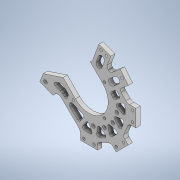
# Autodesk Inventor part: motor_holder_4
Saved by Autodesk Inventor 2020 (Build 240168000, 168)
## iProperties
Created: 2020-03-26
Part Number: motor_holder_4
Material: Generic
Document SubType Name: Modeling
Designer: psrobotics
Density: 1 g/cm^3
Appearance: Default
Author: psrobotics
Autodesk Inventor part; units mm, degrees
(part 1 of 2)
ref_plane "YZ Plane" through (0, 0, 0) normal (1, 0, 0) x (0, 1, 0)
ref_plane "XZ Plane" through (0, 0, 0) normal (0, 1, 0) x (-1, 0, 0)
ref_plane "XY Plane" through (0, 0, 0) normal (0, 0, 1) x (1, 0, 0)
sketch "Sketch1" plane through (0, 0, 0) normal (0, 0, 1) x (1, 0, 0)
  circle A0 centre (-20.1972, 20.1972) radius 3.075 projected
  arc A1 (-10.1972, -33.3775) -> (10.6148, -24.7569) centre (-20.1972, 20.1972) ccw projected
  arc A2 (-70.4, 41.4086) -> (-73.6451, 30.854) centre (-20.1972, 20.1972) ccw projected
  circle A3 centre (-68.634, 68.634) radius 50 projected
  circle A4 centre (-20.1972, 20.1972) radius 54.5
  circle A5 centre (-20.1972, 20.1972) radius 22.5
  circle A6 centre (-68.634, 68.634) radius 53
  point P0 (0, 0)
  point P1 (-15.9632, 74.5325)
  point P2 (-22.4794, 42.5811)
  point P3 (-42.5811, 22.4794)
  point P4 (-74.5325, 15.9632)
  point P5 (-73.6451, 30.854)
  point P6 (-10.1972, -33.3775)
  point P7 (10.6148, -24.7569)
  point P8 (-74.5325, 15.9632)
  dimension "d0" = 109
  dimension "d1" = 45
  dimension "d2" = 106
  constraints: 3 centre point, 3 coincident
  measures "d0" diameter of A4
  measures "d1" diameter of A5
  measures "d2" diameter of A6
extrude "Extrusion1" add sketch "Sketch1" along normal blind 5 contours A0 | A4 A6 A5 A1 | A6 A5
sketch "Sketch2" plane through (0, 0, 5) normal (0, 0, 1) x (1, 0, 0)
  arc A0 (-74.5325, 15.9632) -> (-15.9632, 74.5325) centre (-20.1972, 20.1972) ccw
  circle A1 centre (31.0318, 14.1972) radius 2.075
  circle A2 centre (-26.1972, -31.0318) radius 2.075
  circle A3 centre (-14.1972, -31.0318) radius 2.075
  circle A4 centre (31.0318, 26.1972) radius 2.075
  line L0 (34.8028, 30.1972) -> (27.2607, 30.1972)
  line L1 (27.2607, 10.1972) -> (27.2607, 30.1972)
  arc A5 (20.4317, -6.2895) -> (27.2607, 10.1972) centre (-20.1972, 20.1972) ccw
  line L2 (6.2895, -20.4317) -> (20.4317, -6.2895)
  arc A6 (-10.1972, -27.2607) -> (6.2895, -20.4317) centre (-20.1972, 20.1972) ccw
  line L3 (-30.1972, -27.2607) -> (-10.1972, -27.2607)
  line L4 (-30.1972, -27.2607) -> (-30.1972, -34.8028)
  line L5 (-10.1972, -34.8028) -> (-30.1972, -34.8028)
  line L6 (-10.1972, -33.3775) -> (-10.1972, -34.8028)
  arc A7 (-10.1972, -33.3775) -> (10.6148, -24.7569) centre (-20.1972, 20.1972) ccw
  line L7 (11.6226, -25.7648) -> (10.6148, -24.7569)
  line L8 (25.7648, -11.6226) -> (11.6226, -25.7648)
  line L9 (24.7569, -10.6148) -> (25.7648, -11.6226)
  arc A8 (24.7569, -10.6148) -> (33.3775, 10.1972) centre (-20.1972, 20.1972) ccw
  line L10 (34.8028, 10.1972) -> (33.3775, 10.1972)
  line L11 (34.8028, 30.1972) -> (34.8028, 10.1972)
  circle A9 centre (-10.8666, 70.4743) radius 2.075
  line L12 (-36.782, 65.7734) -> (-41.4086, 70.4)
  arc A10 (-17.5734, 68.6262) -> (-36.782, 65.7734) centre (-20.1972, 20.1972) ccw
  line L13 (-5.9823, 65.5203) -> (-17.5734, 68.6262)
  line L14 (-4.1597, 72.3225) -> (-5.9823, 65.5203)
  line L15 (-15.7508, 75.4283) -> (-4.1597, 72.3225)
  spline S0 degree 3 poles (-17.8978, 74.6487) (-17.5075, 74.6322) (-17.1177, 74.6921) (-16.3809, 74.9587) (-16.0413, 75.1637) (-15.7508, 75.4283) knots 0 0 0 0 0.498547 0.498547 1 1 1 1
  arc A11 (-17.8978, 74.6487) -> (-30.854, 73.6451) centre (-20.1972, 20.1972) ccw
  arc A12 (-30.854, 73.6451) -> (-41.4086, 70.4) centre (-20.1972, 20.1972) ccw
  circle A13 centre (-70.4743, 10.8666) radius 2.075
  line L16 (-70.4, 41.4086) -> (-65.7734, 36.782)
  arc A14 (-70.4, 41.4086) -> (-73.6451, 30.854) centre (-20.1972, 20.1972) ccw
  arc A15 (-73.6451, 30.854) -> (-74.6487, 17.8978) centre (-20.1972, 20.1972) ccw
  spline S1 degree 3 poles (-74.6487, 17.8978) (-74.6321, 17.5052) (-74.6928, 17.1132) (-74.9611, 16.377) (-75.1652, 16.0396) (-75.4283, 15.7508) knots 0 0 0 0 0.501453 0.501453 1 1 1 1
  line L17 (-72.3225, 4.1597) -> (-75.4283, 15.7508)
  line L18 (-65.5203, 5.9823) -> (-72.3225, 4.1597)
  line L19 (-68.6262, 17.5734) -> (-65.5203, 5.9823)
  arc A16 (-65.7734, 36.782) -> (-68.6262, 17.5734) centre (-20.1972, 20.1972) ccw
  line L20 (-75.4283, 15.7508) -> (-68.6262, 17.5734)
  line L21 (-15.7508, 75.4283) -> (-17.5734, 68.6262)
  point P0 (0, 0)
  constraints: 4 end point, 2 perpendicular, 1 other
extrude "Extrusion2" add sketch "Sketch2" against normal up to surface (5 mm away) contours A0 L4 L3 A6 L2 A5 L1 L0 | L6 L5 L4 A0 | A0 L9 L8 L7 | A0 L0 L11 L10 | L17 L20 L19 L18 A0 | A0 L18 L17 | L14 L13 L21 L15 A0 | A0 L15 L14 | A1 | A2 | A3 | A4
sketch "Sketch3" plane through (0, 0, 5) normal (0, 0, 1) x (1, 0, 0)
  circle A0 centre (31.0318, 26.1972) radius 2.075 projected
  circle A1 centre (31.0318, 14.1972) radius 2.075 projected
  circle A2 centre (-14.1972, -31.0318) radius 2.075 projected
  circle A3 centre (-26.1972, -31.0318) radius 2.075 projected
  circle A4 centre (-70.4743, 10.8666) radius 2.075 projected
  circle A5 centre (-10.8666, 70.4743) radius 2.075 projected
  point P0 (0, 0)
hole "Hole1" at (31.0318, 26.1972, 5) at (31.0318, 14.1972, 5) at (-14.1972, -31.0318, 5) at (-26.1972, -31.0318, 5) at (-70.4743, 10.8666, 5) at (-10.8666, 70.4743, 5) direction (0, 0, -1) diameter 4.15 depth 7
sketch "Sketch4" plane through (0, 0, 5) normal (0, 0, 1) x (1, 0, 0)
  circle A0 centre (-20.1972, 20.1972) radius 17.5 projected
  circle A1 centre (-20.1972, 20.1972) radius 22.5
  point P0 (0, 0)
  dimension "d14" = 45
  constraints: 1 centre point, 1 coincident
  measures "d14" diameter of A1
extrude "Extrusion3" cut sketch "Sketch4" against normal blind 10 contours A0 | A1
sketch "Sketch5" plane through (0, 0, 0) normal (0, 0, -1) x (-1, 0, 0)
  arc A0 (22.4794, 42.5811) -> (42.5811, 22.4794) centre (20.1972, 20.1972) ccw projected
  arc A1 (15.6366, 68.1072) -> (22.4794, 42.5811) centre (68.634, 68.634) ccw projected
  line L0 (15.6366, 68.1072) -> (17.5734, 68.6262) projected
  line L1 (17.5734, 68.6262) -> (15.7508, 75.4283) projected
  line L2 (15.7508, 75.4283) -> (4.1597, 72.3225) projected
  line L3 (4.1597, 72.3225) -> (4.1692, 72.287) projected
  arc A2 (4.1692, 72.287) -> (-33.3775, 30.1972) centre (20.1972, 20.1972) ccw projected
  line L4 (-33.3775, 30.1972) -> (-34.8028, 30.1972) projected
  line L5 (-34.8028, 30.1972) -> (-34.8028, 10.1972) projected
  line L6 (-34.8028, 10.1972) -> (-33.3775, 10.1972) projected
  arc A3 (-33.3775, 10.1972) -> (-24.7569, -10.6148) centre (20.1972, 20.1972) ccw projected
  line L7 (-24.7569, -10.6148) -> (-25.7648, -11.6226) projected
  line L8 (-25.7648, -11.6226) -> (-11.6226, -25.7648) projected
  line L9 (-11.6226, -25.7648) -> (-10.6148, -24.7569) projected
  arc A4 (-10.6148, -24.7569) -> (10.1972, -33.3775) centre (20.1972, 20.1972) ccw projected
  line L10 (10.1972, -33.3775) -> (10.1972, -34.8028) projected
  line L11 (10.1972, -34.8028) -> (30.1972, -34.8028) projected
  line L12 (30.1972, -34.8028) -> (30.1972, -33.3775) projected
  arc A5 (30.1972, -33.3775) -> (72.287, 4.1692) centre (20.1972, 20.1972) ccw projected
  line L13 (72.287, 4.1692) -> (72.3225, 4.1597) projected
  line L14 (72.3225, 4.1597) -> (75.4283, 15.7508) projected
  line L15 (75.4283, 15.7508) -> (68.6262, 17.5734) projected
  line L16 (68.6262, 17.5734) -> (68.1072, 15.6366) projected
  arc A6 (42.5811, 22.4794) -> (68.1072, 15.6366) centre (68.634, 68.634) ccw projected
  circle A7 centre (70.4743, 10.8666) radius 2.075 projected
  circle A8 centre (14.1972, -31.0318) radius 2.075 projected
  circle A9 centre (-31.0318, 26.1972) radius 2.075 projected
  circle A10 centre (-31.0318, 14.1972) radius 2.075 projected
  circle A11 centre (26.1972, -31.0318) radius 2.075 projected
  circle A12 centre (10.8666, 70.4743) radius 2.075 projected
  line L17 (72.3225, 4.1597) -> (65.5203, 5.9823) projected
  line L18 (30.1972, -34.8028) -> (30.1972, -5.9562) projected
  line L19 (-5.9562, 30.1972) -> (-34.8028, 30.1972) projected
  line L20 (4.1597, 72.3225) -> (5.9823, 65.5203) projected
  line L21 (20.1972, 20.1972) -> (0, 0)
  line L22 (5.9823, 65.5203) -> (-29.3408, 30.1972)
  line L23 (65.5203, 5.9823) -> (30.1972, -29.3408)
  constraints: 6 end point, 2 parallel, 2 point on line
extrude "Extrusion4" cut sketch "Sketch5" against normal blind 10 contours L20 L22 L19 A2 | A5 L18 L23 L17
sketch "Sketch6" plane through (0, 0, 5) normal (0, 0, 1) x (1, 0, 0)
  circle A0 centre (-70.4743, 10.8666) radius 2.075 projected
  circle A1 centre (-14.1972, -31.0318) radius 2.075 projected
  circle A2 centre (31.0318, 26.1972) radius 2.075 projected
  circle A3 centre (31.0318, 14.1972) radius 2.075 projected
  circle A4 centre (-26.1972, -31.0318) radius 2.075 projected
  circle A5 centre (-10.8666, 70.4743) radius 2.075 projected
  line L0 (34.8028, 30.1972) -> (29.3408, 30.1972) projected
  line L1 (29.3408, 30.1972) -> (-5.9823, 65.5203) projected
  line L2 (-5.9823, 65.5203) -> (-4.1597, 72.3225) projected
  line L3 (-4.1597, 72.3225) -> (-15.7508, 75.4283) projected
  line L4 (-15.7508, 75.4283) -> (-17.5734, 68.6262) projected
  line L5 (-17.5734, 68.6262) -> (-15.6366, 68.1072) projected
  arc A6 (-22.4794, 42.5811) -> (-15.6366, 68.1072) centre (-68.634, 68.634) ccw projected
  arc A7 (-42.5811, 22.4794) -> (-22.4794, 42.5811) centre (-20.1972, 20.1972) ccw projected
  arc A8 (-68.1072, 15.6366) -> (-42.5811, 22.4794) centre (-68.634, 68.634) ccw projected
  line L6 (-68.1072, 15.6366) -> (-68.6262, 17.5734) projected
  line L7 (-68.6262, 17.5734) -> (-75.4283, 15.7508) projected
  line L8 (-75.4283, 15.7508) -> (-72.3225, 4.1597) projected
  line L9 (-72.3225, 4.1597) -> (-65.5203, 5.9823) projected
  line L10 (-65.5203, 5.9823) -> (-30.1972, -29.3408) projected
  line L11 (-30.1972, -29.3408) -> (-30.1972, -34.8028) projected
  line L12 (-30.1972, -34.8028) -> (-10.1972, -34.8028) projected
  line L13 (-10.1972, -34.8028) -> (-10.1972, -33.3775) projected
  arc A9 (-10.1972, -33.3775) -> (10.6148, -24.7569) centre (-20.1972, 20.1972) ccw projected
  line L14 (10.6148, -24.7569) -> (11.6226, -25.7648) projected
  line L15 (11.6226, -25.7648) -> (25.7648, -11.6226) projected
  line L16 (25.7648, -11.6226) -> (24.7569, -10.6148) projected
  arc A10 (24.7569, -10.6148) -> (33.3775, 10.1972) centre (-20.1972, 20.1972) ccw projected
  line L17 (33.3775, 10.1972) -> (34.8028, 10.1972) projected
  line L18 (34.8028, 10.1972) -> (34.8028, 30.1972) projected
  line L19 (-20.1972, 20.1972) -> (-4.2873, 36.1071)
  arc A11 (-42.5811, 22.4794) -> (-22.4794, 42.5811) centre (-20.1972, 20.1972) ccw projected
  line L20 (-20.1972, 20.1972) -> (-36.1071, 4.2873)
  line L21 (-20.1972, 20.1972) -> (0, 0)
  line L22 (-4.2873, 36.1071) -> (-18.7922, 50.612)
  line L23 (-36.1071, 4.2873) -> (-50.612, 18.7922)
  point P0 (-36.1071, 4.2873)
  point P1 (-4.2873, 36.1071)
  constraints: 10 end point, 4 perpendicular, 4 point on circle
extrude "Extrusion5" cut sketch "Sketch6" against normal blind 10 contours L22 A7 A6 | L23 A8 A7
sketch "Sketch7" plane through (0, 0, 5) normal (0, 0, 1) x (1, 0, 0)
  circle A0 centre (-10.8666, 70.4743) radius 2.075 projected
  circle A1 centre (-26.1972, -31.0318) radius 2.075 projected
  circle A2 centre (31.0318, 14.1972) radius 2.075 projected
  circle A3 centre (31.0318, 26.1972) radius 2.075 projected
  circle A4 centre (-14.1972, -31.0318) radius 2.075 projected
  circle A5 centre (-70.4743, 10.8666) radius 2.075 projected
  line L0 (-36.1071, 4.2873) -> (-50.612, 18.7922) projected
  arc A6 (-68.1072, 15.6366) -> (-50.612, 18.7922) centre (-68.634, 68.634) ccw projected
  line L1 (-68.1072, 15.6366) -> (-68.6262, 17.5734) projected
  line L2 (-68.6262, 17.5734) -> (-75.4283, 15.7508) projected
  line L3 (-75.4283, 15.7508) -> (-72.3225, 4.1597) projected
  line L4 (-72.3225, 4.1597) -> (-65.5203, 5.9823) projected
  line L5 (-65.5203, 5.9823) -> (-30.1972, -29.3408) projected
  line L6 (-30.1972, -29.3408) -> (-30.1972, -34.8028) projected
  line L7 (-30.1972, -34.8028) -> (-10.1972, -34.8028) projected
  line L8 (-10.1972, -34.8028) -> (-10.1972, -33.3775) projected
  arc A7 (-10.1972, -33.3775) -> (10.6148, -24.7569) centre (-20.1972, 20.1972) ccw projected
  line L9 (10.6148, -24.7569) -> (11.6226, -25.7648) projected
  line L10 (11.6226, -25.7648) -> (25.7648, -11.6226) projected
  line L11 (25.7648, -11.6226) -> (24.7569, -10.6148) projected
  arc A8 (24.7569, -10.6148) -> (33.3775, 10.1972) centre (-20.1972, 20.1972) ccw projected
  line L12 (33.3775, 10.1972) -> (34.8028, 10.1972) projected
  line L13 (34.8028, 10.1972) -> (34.8028, 30.1972) projected
  line L14 (34.8028, 30.1972) -> (29.3408, 30.1972) projected
  line L15 (29.3408, 30.1972) -> (-5.9823, 65.5203) projected
  line L16 (-5.9823, 65.5203) -> (-4.1597, 72.3225) projected
  line L17 (-4.1597, 72.3225) -> (-15.7508, 75.4283) projected
  line L18 (-15.7508, 75.4283) -> (-17.5734, 68.6262) projected
  line L19 (-17.5734, 68.6262) -> (-15.6366, 68.1072) projected
  arc A9 (-18.7922, 50.612) -> (-15.6366, 68.1072) centre (-68.634, 68.634) ccw projected
  line L20 (-18.7922, 50.612) -> (-4.2873, 36.1071) projected
  arc A10 (-36.1071, 4.2873) -> (-4.2873, 36.1071) centre (-20.1972, 20.1972) ccw projected
  line L21 (-4.1597, 72.3225) -> (-5.9823, 65.5203) projected
  line L22 (-4.1597, 72.3225) -> (34.8028, 30.1972)
  line L23 (-72.3225, 4.1597) -> (-30.1972, -34.8028)
  point P0 (0, 0)
  constraints: 4 end point
extrude "Extrusion6" add sketch "Sketch7" against normal up to surface (5 mm away) contours L4 L5 L6 L23 | L22 L14 L15 L16
sketch "Sketch8" plane through (0, 0, 5) normal (0, 0, 1) x (1, 0, 0)
  circle A0 centre (31.0318, 14.1972) radius 2.075 projected
  circle A1 centre (31.0318, 26.1972) radius 2.075 projected
  circle A2 centre (-10.8666, 70.4743) radius 2.075 projected
  circle A3 centre (-70.4743, 10.8666) radius 2.075 projected
  circle A4 centre (-26.1972, -31.0318) radius 2.075 projected
  circle A5 centre (-14.1972, -31.0318) radius 2.075 projected
  circle A6 centre (-14.1972, -31.0318) radius 2.075 projected
  circle A7 centre (-14.1972, -31.0318) radius 1.5
  circle A8 centre (-26.1972, -31.0318) radius 2.075 projected
  circle A9 centre (-26.1972, -31.0318) radius 1.5
  circle A10 centre (-70.4743, 10.8666) radius 2.075 projected
  circle A11 centre (-70.4743, 10.8666) radius 1.5
  circle A12 centre (31.0318, 14.1972) radius 2.075 projected
  circle A13 centre (31.0318, 14.1972) radius 1.5
  circle A14 centre (31.0318, 26.1972) radius 2.075 projected
  circle A15 centre (31.0318, 26.1972) radius 1.5
  circle A16 centre (-10.8666, 70.4743) radius 2.075 projected
  circle A17 centre (-10.8666, 70.4743) radius 1.5
  point P0 (0, 0)
  dimension "d24" = 3
  dimension "d25" = 3
  dimension "d26" = 3
  dimension "d27" = 3
  dimension "d28" = 3
  dimension "d29" = 3
  constraints: 6 centre point, 6 coincident
  measures "d24" diameter of A7
  measures "d25" diameter of A9
  measures "d26" diameter of A11
  measures "d27" diameter of A13
  measures "d28" diameter of A15
  measures "d29" diameter of A17
extrude "Extrusion7" add sketch "Sketch8" against normal up to surface (5 mm away)
sketch "Sketch9" plane through (0, 0, 5) normal (0, 0, 1) x (1, 0, 0)
  circle A0 centre (-70.4743, 10.8666) radius 1.5 projected
  circle A1 centre (-14.1972, -31.0318) radius 1.5 projected
  circle A2 centre (31.0318, 26.1972) radius 1.5 projected
  circle A3 centre (31.0318, 14.1972) radius 1.5 projected
  circle A4 centre (-26.1972, -31.0318) radius 1.5 projected
  circle A5 centre (-10.8666, 70.4743) radius 1.5 projected
  line L0 (-36.1071, 4.2873) -> (-50.612, 18.7922) projected
  arc A6 (-68.1072, 15.6366) -> (-50.612, 18.7922) centre (-68.634, 68.634) ccw projected
  line L1 (-68.6262, 17.5734) -> (-75.4283, 15.7508) projected
  line L2 (-75.4283, 15.7508) -> (-72.3225, 4.1597) projected
  line L3 (-72.3225, 4.1597) -> (-30.1972, -34.8028) projected
  line L4 (-30.1972, -34.8028) -> (-10.1972, -34.8028) projected
  line L5 (-10.1972, -34.8028) -> (-10.1972, -33.3775) projected
  arc A7 (-10.1972, -33.3775) -> (10.6148, -24.7569) centre (-20.1972, 20.1972) ccw projected
  line L6 (10.6148, -24.7569) -> (11.6226, -25.7648) projected
  line L7 (11.6226, -25.7648) -> (25.7648, -11.6226) projected
  line L8 (25.7648, -11.6226) -> (24.7569, -10.6148) projected
  arc A8 (24.7569, -10.6148) -> (33.3775, 10.1972) centre (-20.1972, 20.1972) ccw projected
  line L9 (33.3775, 10.1972) -> (34.8028, 10.1972) projected
  line L10 (34.8028, 10.1972) -> (34.8028, 30.1972) projected
  line L11 (34.8028, 30.1972) -> (-4.1597, 72.3225) projected
  line L12 (-4.1597, 72.3225) -> (-15.7508, 75.4283) projected
  line L13 (-15.7508, 75.4283) -> (-17.5734, 68.6262) projected
  arc A9 (-18.7922, 50.612) -> (-15.6366, 68.1072) centre (-68.634, 68.634) ccw projected
  line L14 (-18.7922, 50.612) -> (-4.2873, 36.1071) projected
  arc A10 (-36.1071, 4.2873) -> (-4.2873, 36.1071) centre (-20.1972, 20.1972) ccw projected
  circle A11 centre (20.2698, -11.7845) radius 2.075 projected
  circle A12 centre (11.7845, -20.2698) radius 2.075 projected
  line L15 (-68.1072, 15.6366) -> (-68.6262, 17.5734) projected
  line L16 (-17.5734, 68.6262) -> (-15.6366, 68.1072) projected
  point P0 (0, 0)
hole "Hole2" at (20.2698, -11.7845, 5) at (11.7845, -20.2698, 5) direction (0, 0, -1) diameter 3 depth 7
sketch "Sketch10" plane through (0, 0, 5) normal (0, 0, 1) x (1, 0, 0)
  circle A0 centre (20.2698, -11.7845) radius 1.5 projected
  circle A1 centre (11.7845, -20.2698) radius 1.5 projected
  circle A2 centre (-70.4743, 10.8666) radius 1.5 projected
  circle A3 centre (-14.1972, -31.0318) radius 1.5 projected
  circle A4 centre (31.0318, 26.1972) radius 1.5 projected
  circle A5 centre (31.0318, 14.1972) radius 1.5 projected
  circle A6 centre (-26.1972, -31.0318) radius 1.5 projected
  circle A7 centre (-10.8666, 70.4743) radius 1.5 projected
  line L0 (-36.1071, 4.2873) -> (-50.612, 18.7922) projected
  arc A8 (-68.1072, 15.6366) -> (-50.612, 18.7922) centre (-68.634, 68.634) ccw projected
  line L1 (-68.6262, 17.5734) -> (-75.4283, 15.7508) projected
  line L2 (-75.4283, 15.7508) -> (-72.3225, 4.1597) projected
  line L3 (-72.3225, 4.1597) -> (-30.1972, -34.8028) projected
  line L4 (-30.1972, -34.8028) -> (-10.1972, -34.8028) projected
  line L5 (-10.1972, -34.8028) -> (-10.1972, -33.3775) projected
  arc A9 (-10.1972, -33.3775) -> (10.6148, -24.7569) centre (-20.1972, 20.1972) ccw projected
  line L6 (10.6148, -24.7569) -> (11.6226, -25.7648) projected
  line L7 (11.6226, -25.7648) -> (25.7648, -11.6226) projected
  line L8 (25.7648, -11.6226) -> (24.7569, -10.6148) projected
  arc A10 (24.7569, -10.6148) -> (33.3775, 10.1972) centre (-20.1972, 20.1972) ccw projected
  line L9 (33.3775, 10.1972) -> (34.8028, 10.1972) projected
  line L10 (34.8028, 10.1972) -> (34.8028, 30.1972) projected
  line L11 (34.8028, 30.1972) -> (-4.1597, 72.3225) projected
  line L12 (-4.1597, 72.3225) -> (-15.7508, 75.4283) projected
  line L13 (-15.7508, 75.4283) -> (-17.5734, 68.6262) projected
  arc A11 (-18.7922, 50.612) -> (-15.6366, 68.1072) centre (-68.634, 68.634) ccw projected
  line L14 (-18.7922, 50.612) -> (-4.2873, 36.1071) projected
  arc A12 (-36.1071, 4.2873) -> (-4.2873, 36.1071) centre (-20.1972, 20.1972) ccw projected
  line L15 (33.3775, 10.1972) -> (26.3775, 10.1972)
  line L16 (24.7569, -10.6148) -> (19.8072, -5.665)
  arc A13 (-10.1972, -33.3775) -> (10.6148, -24.7569) centre (-20.1972, 20.1972) ccw projected
  line L17 (10.6148, -24.7569) -> (5.665, -19.8072)
  line L18 (-10.1972, -33.3775) -> (-10.1972, -26.3775)
  line L19 (10.6148, -24.7569) -> (11.6226, -25.7648) projected
  line L20 (26.3775, 10.1972) -> (19.8072, -5.665)
  line L21 (5.665, -19.8072) -> (-10.1972, -26.3775)
  line L22 (-68.1072, 15.6366) -> (-68.6262, 17.5734) projected
  line L23 (-17.5734, 68.6262) -> (-15.6366, 68.1072) projected
  point P0 (0, 0)
  dimension "d39" = 7
  dimension "d40" = 7
  dimension "d41" = 7
  dimension "d42" = 7
  constraints: 12 end point, 2 collinear, 1 horizontal, 1 vertical
  measures "d39" distance of L9.start L15.end
  measures "d40" distance of L8.end L16.end
  measures "d41" distance of L6.start L17.end
  measures "d42" distance of L5.end L18.end
extrude "Extrusion8" cut sketch "Sketch10" against normal blind 10 contours L18 L21 L17 A9 | A10 L16 L20 L15
sketch "Sketch11" plane through (0, 0, 5) normal (0, 0, 1) x (1, 0, 0)
  line L0 (5.665, -19.8072) -> (11.6226, -25.7648) projected
  line L1 (11.6226, -25.7648) -> (25.7648, -11.6226) projected
  line L2 (25.7648, -11.6226) -> (19.8072, -5.665) projected
  line L3 (19.8072, -5.665) -> (26.3775, 10.1972) projected
  line L4 (26.3775, 10.1972) -> (34.8028, 10.1972) projected
  line L5 (34.8028, 10.1972) -> (34.8028, 30.1972) projected
  line L6 (34.8028, 30.1972) -> (-4.1597, 72.3225) projected
  line L7 (-4.1597, 72.3225) -> (-15.7508, 75.4283) projected
  line L8 (-15.7508, 75.4283) -> (-17.5734, 68.6262) projected
  arc A0 (-68.1072, 15.6366) -> (-50.612, 18.7922) centre (-68.634, 68.634) ccw projected
  line L9 (-18.7922, 50.612) -> (-4.2873, 36.1071) projected
  arc A1 (-36.1071, 4.2873) -> (-4.2873, 36.1071) centre (-20.1972, 20.1972) ccw projected
  line L10 (-36.1071, 4.2873) -> (-50.612, 18.7922) projected
  arc A2 (-18.7922, 50.612) -> (-15.6366, 68.1072) centre (-68.634, 68.634) ccw projected
  line L11 (-68.6262, 17.5734) -> (-75.4283, 15.7508) projected
  line L12 (-75.4283, 15.7508) -> (-72.3225, 4.1597) projected
  line L13 (-72.3225, 4.1597) -> (-30.1972, -34.8028) projected
  line L14 (-30.1972, -34.8028) -> (-10.1972, -34.8028) projected
  line L15 (-10.1972, -34.8028) -> (-10.1972, -26.3775) projected
  line L16 (-10.1972, -26.3775) -> (5.665, -19.8072) projected
  circle A3 centre (20.2698, -11.7845) radius 1.5 projected
  circle A4 centre (11.7845, -20.2698) radius 1.5 projected
  circle A5 centre (-70.4743, 10.8666) radius 1.5 projected
  circle A6 centre (-14.1972, -31.0318) radius 1.5 projected
  circle A7 centre (31.0318, 26.1972) radius 1.5 projected
  circle A8 centre (31.0318, 14.1972) radius 1.5 projected
  circle A9 centre (-26.1972, -31.0318) radius 1.5 projected
  circle A10 centre (-10.8666, 70.4743) radius 1.5 projected
  line L17 (34.8028, 30.1972) -> (-4.1597, 72.3225) projected
  line L18 (-4.1597, 72.3225) -> (-6.7479, 62.6632)
  line L19 (34.8028, 10.1972) -> (34.8028, 30.1972) projected
  line L20 (34.8028, 30.1972) -> (24.8028, 30.1972)
  line L21 (-4.1597, 72.3225) -> (-15.7508, 75.4283) projected
  line L22 (-6.7479, 62.6632) -> (24.8028, 30.1972)
  line L23 (-17.5734, 68.6262) -> (-15.6366, 68.1072) projected
  line L24 (-68.1072, 15.6366) -> (-68.6262, 17.5734) projected
  point P0 (0, 0)
  dimension "d45" = 10
  dimension "d46" = 10
  constraints: 6 end point, 2 perpendicular
  measures "d45" distance of L6.end L18.end
  measures "d46" distance of L5.end L20.end
extrude "Extrusion9" cut sketch "Sketch11" against normal blind 10 contours L20 L22 L18 L6
sketch "Sketch12" plane through (0, 0, 5) normal (0, 0, 1) x (1, 0, 0)
  circle A0 centre (-10.8666, 70.4743) radius 1.5 projected
  circle A1 centre (-26.1972, -31.0318) radius 1.5 projected
  circle A2 centre (31.0318, 14.1972) radius 1.5 projected
  circle A3 centre (31.0318, 26.1972) radius 1.5 projected
  circle A4 centre (-14.1972, -31.0318) radius 1.5 projected
  circle A5 centre (-70.4743, 10.8666) radius 1.5 projected
  circle A6 centre (11.7845, -20.2698) radius 1.5 projected
  circle A7 centre (20.2698, -11.7845) radius 1.5 projected
  line L0 (34.8028, 30.1972) -> (24.8028, 30.1972) projected
  line L1 (24.8028, 30.1972) -> (-6.7479, 62.6632) projected
  line L2 (-6.7479, 62.6632) -> (-4.1597, 72.3225) projected
  line L3 (-4.1597, 72.3225) -> (-15.7508, 75.4283) projected
  line L4 (-15.7508, 75.4283) -> (-17.5734, 68.6262) projected
  arc A8 (-68.1072, 15.6366) -> (-50.612, 18.7922) centre (-68.634, 68.634) ccw projected
  line L5 (-18.7922, 50.612) -> (-4.2873, 36.1071) projected
  arc A9 (-36.1071, 4.2873) -> (-4.2873, 36.1071) centre (-20.1972, 20.1972) ccw projected
  line L6 (-36.1071, 4.2873) -> (-50.612, 18.7922) projected
  arc A10 (-18.7922, 50.612) -> (-15.6366, 68.1072) centre (-68.634, 68.634) ccw projected
  line L7 (-68.6262, 17.5734) -> (-75.4283, 15.7508) projected
  line L8 (-75.4283, 15.7508) -> (-72.3225, 4.1597) projected
  line L9 (-72.3225, 4.1597) -> (-30.1972, -34.8028) projected
  line L10 (-30.1972, -34.8028) -> (-10.1972, -34.8028) projected
  line L11 (-10.1972, -34.8028) -> (-10.1972, -26.3775) projected
  line L12 (-10.1972, -26.3775) -> (5.665, -19.8072) projected
  line L13 (5.665, -19.8072) -> (11.6226, -25.7648) projected
  line L14 (11.6226, -25.7648) -> (25.7648, -11.6226) projected
  line L15 (25.7648, -11.6226) -> (19.8072, -5.665) projected
  line L16 (19.8072, -5.665) -> (26.3775, 10.1972) projected
  line L17 (26.3775, 10.1972) -> (34.8028, 10.1972) projected
  line L18 (34.8028, 10.1972) -> (34.8028, 30.1972) projected
  line L19 (-72.3225, 4.1597) -> (-62.6632, 6.7479)
  line L20 (-10.1972, -34.8028) -> (-30.1972, -34.8028) projected
  line L21 (-30.1972, -34.8028) -> (-30.1972, -24.8028)
  line L22 (-75.4283, 15.7508) -> (-72.3225, 4.1597) projected
  line L23 (-62.6632, 6.7479) -> (-30.1972, -24.8028)
  line L24 (-17.5734, 68.6262) -> (-15.6366, 68.1072) projected
  line L25 (-68.1072, 15.6366) -> (-68.6262, 17.5734) projected
  point P0 (0, 0)
  dimension "d49" = 10
  dimension "d50" = 10
  constraints: 6 end point, 2 perpendicular
  measures "d49" distance of L8.end L19.end
  measures "d50" distance of L9.end L21.end
extrude "Extrusion10" cut sketch "Sketch12" against normal blind 10 contours L9 L19 L23 L21
sketch "Sketch13" plane through (0, 0, 5) normal (0, 0, 1) x (1, 0, 0)
  circle A0 centre (-1.8124, 1.8124) radius 2.075 projected
  circle A1 centre (-38.4172, 1.8124) radius 2.075 projected
  circle A2 centre (-1.8124, 38.4172) radius 2.075 projected
  point P0 (0, 0)
hole "Hole3" at (-1.8124, 1.8124, 5) at (-38.4172, 1.8124, 5) at (-1.8124, 38.4172, 5) direction (0, 0, -1) diameter 3 depth 7
sketch "Sketch14" plane through (0, 0, 5) normal (0, 0, 1) x (1, 0, 0)
  arc A0 (-36.1071, 4.2873) -> (-4.2873, 36.1071) centre (-20.1972, 20.1972) ccw projected
  circle A1 centre (-20.1972, 20.1972) radius 30
  circle A2 centre (-20.1972, 20.1972) radius 42.5
  line L0 (-20.1972, 20.1972) -> (9.8549, -9.8549)
  circle A3 centre (-1.8124, 1.8124) radius 1.5 projected
  line L1 (1.016, -1.016) -> (4.5836, -14.3305)
  line L2 (1.016, -1.016) -> (14.3305, -4.5836)
  point P0 (0, 0)
  dimension "d61" = 60
  dimension "d62" = 85
  dimension "d63" = 30
  dimension "d64" = 30
  constraints: 6 end point, 3 point on circle, 2 coincident, 2 point on line, 1 centre point, 3 other
  measures "d62" diameter of A2
  measures "d63" angle of L1 L0
  measures "d64" angle of L2 L0
extrude "Extrusion11" cut sketch "Sketch14" against normal blind 10 contours L2 A2 L0 | L0 A2 L1
pattern_circular "Circular Pattern1" count 3 over 48 about axis through (-20.1972, 20.1972, 5) along (0, 0, -1) of "Extrusion11"
pattern_circular "Circular Pattern2" count 3 over 48 about axis through (-20.1972, 20.1972, 5) along (0, 0, 1) of "Extrusion11"
fillet "Fillet3" radius 2 3 edges at (9.7617, 21.7673, 2.5) (22.0435, 15.5094, 2.5) (21.3221, 29.2747, 2.5)
pattern_circular "Circular Pattern3" count 5 over 96 about axis through (-20.1972, 20.1972, 5) along (0, 0, -1) of "Fillet3"
sketch "Sketch15" plane through (0, 0, 5) normal (0, 0, 1) x (1, 0, 0)
  arc A0 (22.272, 18.5798) -> (21.8703, 26.245) centre (-20.1972, 20.1972) ccw projected
  arc A1 (19.3655, 16.8739) -> (22.272, 18.5798) centre (20.2735, 18.6559) ccw projected
  line L0 (19.3655, 16.8739) -> (12.8482, 20.1946) projected
  arc A2 (12.6669, 23.6539) -> (12.8482, 20.1946) centre (13.7562, 21.9766) ccw projected
  line L1 (12.6669, 23.6539) -> (18.8014, 27.6377) projected
  arc A3 (21.8703, 26.245) -> (18.8014, 27.6377) centre (19.8907, 25.9604) ccw projected
  arc A4 (17.9425, 1.4458) -> (20.6932, 8.6117) centre (-20.1972, 20.1972) ccw projected
  arc A5 (14.5934, 1.0696) -> (17.9425, 1.4458) centre (16.1477, 2.3282) ccw projected
  line L2 (14.5934, 1.0696) -> (9.9903, 6.754) projected
  arc A6 (11.2317, 9.988) -> (9.9903, 6.754) centre (11.5446, 8.0127) ccw projected
  line L3 (11.2317, 9.988) -> (18.4561, 11.1323) projected
  arc A7 (20.6932, 8.6117) -> (18.4561, 11.1323) centre (18.769, 9.1569) ccw projected
  arc A8 (-26.245, -21.8703) -> (-18.5798, -22.272) centre (-20.1972, 20.1972) ccw projected
  arc A9 (-27.6377, -18.8014) -> (-26.245, -21.8703) centre (-25.9604, -19.8907) ccw projected
  line L4 (-27.6377, -18.8014) -> (-23.6539, -12.6669) projected
  arc A10 (-20.1946, -12.8482) -> (-23.6539, -12.6669) centre (-21.9766, -13.7562) ccw projected
  line L5 (-20.1946, -12.8482) -> (-16.8739, -19.3655) projected
  arc A11 (-18.5798, -22.272) -> (-16.8739, -19.3655) centre (-18.6559, -20.2735) ccw projected
  arc A12 (-8.6117, -20.6932) -> (-1.4458, -17.9425) centre (-20.1972, 20.1972) ccw projected
  arc A13 (-11.1323, -18.4561) -> (-8.6117, -20.6932) centre (-9.1569, -18.769) ccw projected
  line L6 (-11.1323, -18.4561) -> (-9.988, -11.2317) projected
  arc A14 (-6.754, -9.9903) -> (-9.988, -11.2317) centre (-8.0127, -11.5446) ccw projected
  line L7 (-6.754, -9.9903) -> (-1.0696, -14.5934) projected
  arc A15 (-1.4458, -17.9425) -> (-1.0696, -14.5934) centre (-2.3282, -16.1477) ccw projected
  arc A16 (7.0183, -12.4458) -> (12.4458, -7.0183) centre (-20.1972, 20.1972) ccw projected
  arc A17 (3.8057, -11.4273) -> (7.0183, -12.4458) centre (5.7376, -10.9097) ccw projected
  line L8 (3.8057, -11.4273) -> (1.9126, -4.3621) projected
  arc A18 (4.3621, -1.9126) -> (1.9126, -4.3621) centre (3.8444, -3.8444) ccw projected
  line L9 (4.3621, -1.9126) -> (11.4273, -3.8057) projected
  arc A19 (12.4458, -7.0183) -> (11.4273, -3.8057) centre (10.9097, -5.7376) ccw projected
  circle A20 centre (-38.4172, 1.8124) radius 1.5 projected
  circle A21 centre (-1.8124, 1.8124) radius 1.5 projected
  circle A22 centre (-1.8124, 38.4172) radius 1.5 projected
  line L10 (-18.7922, 50.612) -> (-4.2873, 36.1071) projected
  arc A23 (-36.1071, 4.2873) -> (-4.2873, 36.1071) centre (-20.1972, 20.1972) ccw projected
  line L11 (-36.1071, 4.2873) -> (-50.612, 18.7922) projected
  arc A24 (-68.1072, 15.6366) -> (-50.612, 18.7922) centre (-68.634, 68.634) ccw projected
  line L12 (-68.6262, 17.5734) -> (-75.4283, 15.7508) projected
  line L13 (-75.4283, 15.7508) -> (-72.3225, 4.1597) projected
  line L14 (-72.3225, 4.1597) -> (-62.6632, 6.7479) projected
  line L15 (-62.6632, 6.7479) -> (-30.1972, -24.8028) projected
  line L16 (-30.1972, -24.8028) -> (-30.1972, -34.8028) projected
  line L17 (-30.1972, -34.8028) -> (-10.1972, -34.8028) projected
  line L18 (-10.1972, -34.8028) -> (-10.1972, -26.3775) projected
  line L19 (-10.1972, -26.3775) -> (5.665, -19.8072) projected
  line L20 (5.665, -19.8072) -> (11.6226, -25.7648) projected
  line L21 (11.6226, -25.7648) -> (25.7648, -11.6226) projected
  line L22 (25.7648, -11.6226) -> (19.8072, -5.665) projected
  line L23 (19.8072, -5.665) -> (26.3775, 10.1972) projected
  line L24 (26.3775, 10.1972) -> (34.8028, 10.1972) projected
  line L25 (34.8028, 10.1972) -> (34.8028, 30.1972) projected
  line L26 (34.8028, 30.1972) -> (24.8028, 30.1972) projected
  line L27 (24.8028, 30.1972) -> (-6.7479, 62.6632) projected
  line L28 (-6.7479, 62.6632) -> (-4.1597, 72.3225) projected
  line L29 (-4.1597, 72.3225) -> (-15.7508, 75.4283) projected
  line L30 (-15.7508, 75.4283) -> (-17.5734, 68.6262) projected
  arc A25 (-18.7922, 50.612) -> (-15.6366, 68.1072) centre (-68.634, 68.634) ccw projected
  circle A26 centre (20.2698, -11.7845) radius 1.5 projected
  circle A27 centre (11.7845, -20.2698) radius 1.5 projected
  circle A28 centre (-70.4743, 10.8666) radius 1.5 projected
  circle A29 centre (-14.1972, -31.0318) radius 1.5 projected
  circle A30 centre (31.0318, 26.1972) radius 1.5 projected
  circle A31 centre (31.0318, 14.1972) radius 1.5 projected
  circle A32 centre (-26.1972, -31.0318) radius 1.5 projected
  circle A33 centre (-10.8666, 70.4743) radius 1.5 projected
  arc A34 (12.6669, 23.6539) -> (12.8482, 20.1946) centre (13.7562, 21.9766) ccw projected
  arc A35 (11.2317, 9.988) -> (9.9903, 6.754) centre (11.5446, 8.0127) ccw projected
  line L31 (13.7562, 21.9766) -> (11.5446, 8.0127)
  line L32 (11.5446, 8.0127) -> (3.8444, -3.8444)
  line L33 (3.8444, -3.8444) -> (-8.0127, -11.5446)
  line L34 (-8.0127, -11.5446) -> (-21.9766, -13.7562)
  circle A36 centre (12.6504, 14.9946) radius 2.075
  circle A37 centre (7.6945, 2.0841) radius 2.075
  circle A38 centre (-2.0841, -7.6945) radius 2.075
  circle A39 centre (-14.9946, -12.6504) radius 2.075
  line L35 (-17.5734, 68.6262) -> (-15.6366, 68.1072) projected
  line L36 (-68.1072, 15.6366) -> (-68.6262, 17.5734) projected
  point P0 (0, 0)
  dimension "d77" = 4.15
  dimension "d78" = 4.15
  dimension "d79" = 4.15
  dimension "d80" = 4.15
  constraints: 8 end point, 4 centre point, 4 midpoint
  measures "d77" diameter of A36
  measures "d78" diameter of A37
  measures "d79" diameter of A38
  measures "d80" diameter of A39
extrude "Extrusion12" cut sketch "Sketch15" against normal blind 10 contours A36 L31 | L31 A36 | A37 L32 | L32 A37 | A38 L33 | L33 A38 | A39 L34 | L34 A39
fillet "Fillet5" radius 4 4 edges at (26.3775, 10.1972, 2.5) (19.8072, -5.665, 2.5) (5.665, -19.8072, 2.5) (-10.1972, -26.3775, 2.5)
sketch "Sketch17" plane through (0, 0, 0) normal (0, 0, -1) x (-1, 0, 0)
  circle A0 centre (2.0841, -7.6945) radius 2.075 projected
  circle A1 centre (-7.6945, 2.0841) radius 2.075 projected
  circle A2 centre (14.9946, -12.6504) radius 2.075 projected
  circle A3 centre (-12.6504, 14.9946) radius 2.075 projected
  arc A4 (-21.8703, 26.245) -> (-22.272, 18.5798) centre (20.1972, 20.1972) ccw projected
  arc A5 (-18.8014, 27.6377) -> (-21.8703, 26.245) centre (-19.8907, 25.9604) ccw projected
  line L0 (-18.8014, 27.6377) -> (-12.6669, 23.6539) projected
  arc A6 (-12.8482, 20.1946) -> (-12.6669, 23.6539) centre (-13.7562, 21.9766) ccw projected
  line L1 (-12.8482, 20.1946) -> (-19.3655, 16.8739) projected
  arc A7 (-22.272, 18.5798) -> (-19.3655, 16.8739) centre (-20.2735, 18.6559) ccw projected
  arc A8 (-20.6932, 8.6117) -> (-17.9425, 1.4458) centre (20.1972, 20.1972) ccw projected
  arc A9 (-18.4561, 11.1323) -> (-20.6932, 8.6117) centre (-18.769, 9.1569) ccw projected
  line L2 (-18.4561, 11.1323) -> (-11.2317, 9.988) projected
  arc A10 (-9.9903, 6.754) -> (-11.2317, 9.988) centre (-11.5446, 8.0127) ccw projected
  line L3 (-9.9903, 6.754) -> (-14.5934, 1.0696) projected
  arc A11 (-17.9425, 1.4458) -> (-14.5934, 1.0696) centre (-16.1477, 2.3282) ccw projected
  arc A12 (18.5798, -22.272) -> (26.245, -21.8703) centre (20.1972, 20.1972) ccw projected
  arc A13 (16.8739, -19.3655) -> (18.5798, -22.272) centre (18.6559, -20.2735) ccw projected
  line L4 (16.8739, -19.3655) -> (20.1946, -12.8482) projected
  arc A14 (23.6539, -12.6669) -> (20.1946, -12.8482) centre (21.9766, -13.7562) ccw projected
  line L5 (23.6539, -12.6669) -> (27.6377, -18.8014) projected
  arc A15 (26.245, -21.8703) -> (27.6377, -18.8014) centre (25.9604, -19.8907) ccw projected
  arc A16 (1.4458, -17.9425) -> (8.6117, -20.6932) centre (20.1972, 20.1972) ccw projected
  arc A17 (1.0696, -14.5934) -> (1.4458, -17.9425) centre (2.3282, -16.1477) ccw projected
  line L6 (1.0696, -14.5934) -> (6.754, -9.9903) projected
  arc A18 (9.988, -11.2317) -> (6.754, -9.9903) centre (8.0127, -11.5446) ccw projected
  line L7 (9.988, -11.2317) -> (11.1323, -18.4561) projected
  arc A19 (8.6117, -20.6932) -> (11.1323, -18.4561) centre (9.1569, -18.769) ccw projected
  arc A20 (-12.4458, -7.0183) -> (-7.0183, -12.4458) centre (20.1972, 20.1972) ccw projected
  arc A21 (-11.4273, -3.8057) -> (-12.4458, -7.0183) centre (-10.9097, -5.7376) ccw projected
  line L8 (-11.4273, -3.8057) -> (-4.3621, -1.9126) projected
  arc A22 (-1.9126, -4.3621) -> (-4.3621, -1.9126) centre (-3.8444, -3.8444) ccw projected
  line L9 (-1.9126, -4.3621) -> (-3.8057, -11.4273) projected
  arc A23 (-7.0183, -12.4458) -> (-3.8057, -11.4273) centre (-5.7376, -10.9097) ccw projected
  circle A24 centre (38.4172, 1.8124) radius 1.5 projected
  circle A25 centre (1.8124, 1.8124) radius 1.5 projected
  circle A26 centre (1.8124, 38.4172) radius 1.5 projected
  circle A27 centre (10.8666, 70.4743) radius 1.5 projected
  circle A28 centre (26.1972, -31.0318) radius 1.5 projected
  circle A29 centre (-31.0318, 14.1972) radius 1.5 projected
  circle A30 centre (-31.0318, 26.1972) radius 1.5 projected
  circle A31 centre (14.1972, -31.0318) radius 1.5 projected
  circle A32 centre (70.4743, 10.8666) radius 1.5 projected
  circle A33 centre (-11.7845, -20.2698) radius 1.5 projected
  circle A34 centre (-20.2698, -11.7845) radius 1.5 projected
  line L10 (30.1972, -34.8028) -> (30.1972, -24.8028) projected
  line L11 (30.1972, -24.8028) -> (62.6632, 6.7479) projected
  line L12 (62.6632, 6.7479) -> (72.3225, 4.1597) projected
  line L13 (72.3225, 4.1597) -> (75.4283, 15.7508) projected
  line L14 (75.4283, 15.7508) -> (68.6262, 17.5734) projected
  line L15 (68.6262, 17.5734) -> (68.1072, 15.6366) projected
  arc A35 (50.612, 18.7922) -> (68.1072, 15.6366) centre (68.634, 68.634) ccw projected
  line L16 (50.612, 18.7922) -> (36.1071, 4.2873) projected
  arc A36 (4.2873, 36.1071) -> (36.1071, 4.2873) centre (20.1972, 20.1972) ccw projected
  line L17 (4.2873, 36.1071) -> (18.7922, 50.612) projected
  arc A37 (15.6366, 68.1072) -> (18.7922, 50.612) centre (68.634, 68.634) ccw projected
  line L18 (15.6366, 68.1072) -> (17.5734, 68.6262) projected
  line L19 (17.5734, 68.6262) -> (15.7508, 75.4283) projected
  line L20 (15.7508, 75.4283) -> (4.1597, 72.3225) projected
  line L21 (4.1597, 72.3225) -> (6.7479, 62.6632) projected
  line L22 (6.7479, 62.6632) -> (-24.8028, 30.1972) projected
  line L23 (-24.8028, 30.1972) -> (-34.8028, 30.1972) projected
  line L24 (-34.8028, 30.1972) -> (-34.8028, 10.1972) projected
  line L25 (-34.8028, 10.1972) -> (-29.0502, 10.1972) projected
  arc A38 (-25.3547, 7.7279) -> (-29.0502, 10.1972) centre (-29.0502, 6.1972) ccw projected
  line L26 (-25.3547, 7.7279) -> (-20.83, -3.1958) projected
  arc A39 (-21.6971, -7.5549) -> (-20.83, -3.1958) centre (-24.5255, -4.7265) ccw projected
  line L27 (-21.6971, -7.5549) -> (-25.7648, -11.6226) projected
  line L28 (-25.7648, -11.6226) -> (-11.6226, -25.7648) projected
  line L29 (-11.6226, -25.7648) -> (-7.5549, -21.6971) projected
  arc A40 (-3.1958, -20.83) -> (-7.5549, -21.6971) centre (-4.7265, -24.5255) ccw projected
  line L30 (-3.1958, -20.83) -> (7.7279, -25.3547) projected
  arc A41 (10.1972, -29.0502) -> (7.7279, -25.3547) centre (6.1972, -29.0502) ccw projected
  line L31 (10.1972, -29.0502) -> (10.1972, -34.8028) projected
  line L32 (10.1972, -34.8028) -> (30.1972, -34.8028) projected
  line L33 (18.7922, 50.612) -> (6.7479, 62.6632)
  line L34 (50.612, 18.7922) -> (62.6632, 6.7479)
  point P0 (0, 0)
  constraints: 4 end point
extrude "Extrusion14" cut sketch "Sketch17" against normal blind 10 contours L34 A35 L15 L14 L13 L12 | L33 L21 L20 L19 L18 A37
sketch "Sketch18" plane through (0, 0, 0) normal (0, 0, -1) x (-1, 0, 0)
  circle A0 centre (71.2839, 4.1003) radius 2.05 projected
  line L0 (78.6856, -1.0442) -> (73.9192, 11.0505) projected
  line L1 (73.9192, 11.0505) -> (67.4066, 8.4839) projected
  line L2 (67.4066, 8.4839) -> (61.7695, -4.4861) projected
  line L3 (61.7695, -4.4861) -> (77.5856, 1.7469) projected
  line L4 (73.9192, 11.0505) -> (77.5856, 1.7469)
  line L5 (18.7922, 50.612) -> (6.7479, 62.6632) projected
  line L6 (6.7479, 62.6632) -> (-24.8028, 30.1972) projected
  line L7 (-24.8028, 30.1972) -> (-34.8028, 30.1972) projected
  line L8 (-34.8028, 30.1972) -> (-34.8028, 10.1972) projected
  line L9 (-34.8028, 10.1972) -> (-29.0502, 10.1972) projected
  arc A1 (-25.3547, 7.7279) -> (-29.0502, 10.1972) centre (-29.0502, 6.1972) ccw projected
  line L10 (-25.3547, 7.7279) -> (-20.83, -3.1958) projected
  arc A2 (-21.6971, -7.5549) -> (-20.83, -3.1958) centre (-24.5255, -4.7265) ccw projected
  line L11 (-21.6971, -7.5549) -> (-25.7648, -11.6226) projected
  line L12 (-25.7648, -11.6226) -> (-11.6226, -25.7648) projected
  line L13 (-11.6226, -25.7648) -> (-7.5549, -21.6971) projected
  arc A3 (-3.1958, -20.83) -> (-7.5549, -21.6971) centre (-4.7265, -24.5255) ccw projected
  line L14 (-3.1958, -20.83) -> (7.7279, -25.3547) projected
  arc A4 (10.1972, -29.0502) -> (7.7279, -25.3547) centre (6.1972, -29.0502) ccw projected
  line L15 (10.1972, -29.0502) -> (10.1972, -34.8028) projected
  line L16 (10.1972, -34.8028) -> (30.1972, -34.8028) projected
  line L17 (30.1972, -34.8028) -> (30.1972, -24.8028) projected
  line L18 (30.1972, -24.8028) -> (62.6632, 6.7479) projected
  line L19 (62.6632, 6.7479) -> (50.612, 18.7922) projected
  line L20 (50.612, 18.7922) -> (36.1071, 4.2873) projected
  arc A5 (4.2873, 36.1071) -> (36.1071, 4.2873) centre (20.1972, 20.1972) ccw projected
  line L21 (4.2873, 36.1071) -> (18.7922, 50.612) projected
  circle A6 centre (2.0841, -7.6945) radius 2.075 projected
  circle A7 centre (-7.6945, 2.0841) radius 2.075 projected
  circle A8 centre (14.9946, -12.6504) radius 2.075 projected
  circle A9 centre (-12.6504, 14.9946) radius 2.075 projected
  arc A10 (-21.8703, 26.245) -> (-22.272, 18.5798) centre (20.1972, 20.1972) ccw projected
  arc A11 (-18.8014, 27.6377) -> (-21.8703, 26.245) centre (-19.8907, 25.9604) ccw projected
  line L22 (-18.8014, 27.6377) -> (-12.6669, 23.6539) projected
  arc A12 (-12.8482, 20.1946) -> (-12.6669, 23.6539) centre (-13.7562, 21.9766) ccw projected
  line L23 (-12.8482, 20.1946) -> (-19.3655, 16.8739) projected
  arc A13 (-22.272, 18.5798) -> (-19.3655, 16.8739) centre (-20.2735, 18.6559) ccw projected
  arc A14 (-20.6932, 8.6117) -> (-17.9425, 1.4458) centre (20.1972, 20.1972) ccw projected
  arc A15 (-18.4561, 11.1323) -> (-20.6932, 8.6117) centre (-18.769, 9.1569) ccw projected
  line L24 (-18.4561, 11.1323) -> (-11.2317, 9.988) projected
  arc A16 (-9.9903, 6.754) -> (-11.2317, 9.988) centre (-11.5446, 8.0127) ccw projected
  line L25 (-9.9903, 6.754) -> (-14.5934, 1.0696) projected
  arc A17 (-17.9425, 1.4458) -> (-14.5934, 1.0696) centre (-16.1477, 2.3282) ccw projected
  arc A18 (18.5798, -22.272) -> (26.245, -21.8703) centre (20.1972, 20.1972) ccw projected
  arc A19 (16.8739, -19.3655) -> (18.5798, -22.272) centre (18.6559, -20.2735) ccw projected
  line L26 (16.8739, -19.3655) -> (20.1946, -12.8482) projected
  arc A20 (23.6539, -12.6669) -> (20.1946, -12.8482) centre (21.9766, -13.7562) ccw projected
  line L27 (23.6539, -12.6669) -> (27.6377, -18.8014) projected
  arc A21 (26.245, -21.8703) -> (27.6377, -18.8014) centre (25.9604, -19.8907) ccw projected
  arc A22 (1.4458, -17.9425) -> (8.6117, -20.6932) centre (20.1972, 20.1972) ccw projected
  arc A23 (1.0696, -14.5934) -> (1.4458, -17.9425) centre (2.3282, -16.1477) ccw projected
  line L28 (1.0696, -14.5934) -> (6.754, -9.9903) projected
  arc A24 (9.988, -11.2317) -> (6.754, -9.9903) centre (8.0127, -11.5446) ccw projected
  line L29 (9.988, -11.2317) -> (11.1323, -18.4561) projected
  arc A25 (8.6117, -20.6932) -> (11.1323, -18.4561) centre (9.1569, -18.769) ccw projected
  arc A26 (-12.4458, -7.0183) -> (-7.0183, -12.4458) centre (20.1972, 20.1972) ccw projected
  arc A27 (-11.4273, -3.8057) -> (-12.4458, -7.0183) centre (-10.9097, -5.7376) ccw projected
  line L30 (-11.4273, -3.8057) -> (-4.3621, -1.9126) projected
  arc A28 (-1.9126, -4.3621) -> (-4.3621, -1.9126) centre (-3.8444, -3.8444) ccw projected
  line L31 (-1.9126, -4.3621) -> (-3.8057, -11.4273) projected
  arc A29 (-7.0183, -12.4458) -> (-3.8057, -11.4273) centre (-5.7376, -10.9097) ccw projected
  circle A30 centre (38.4172, 1.8124) radius 1.5 projected
  circle A31 centre (1.8124, 1.8124) radius 1.5 projected
  circle A32 centre (1.8124, 38.4172) radius 1.5 projected
  circle A33 centre (26.1972, -31.0318) radius 1.5 projected
  circle A34 centre (-31.0318, 14.1972) radius 1.5 projected
  circle A35 centre (-31.0318, 26.1972) radius 1.5 projected
  circle A36 centre (14.1972, -31.0318) radius 1.5 projected
  circle A37 centre (-11.7845, -20.2698) radius 1.5 projected
  circle A38 centre (-20.2698, -11.7845) radius 1.5 projected
  line L32 (50.612, 18.7922) -> (62.6632, 6.7479) projected
  line L33 (73.9192, 11.0505) -> (50.612, 18.7922)
  line L34 (61.7695, -4.4861) -> (56.5889, 0.8448)
  line L35 (30.1972, -24.8028) -> (62.6632, 6.7479) projected
  line L36 (62.8695, -7.2772) -> (78.6856, -1.0442) projected
  line L37 (61.7695, -4.4861) -> (62.8695, -7.2772) projected
  point P0 (0, 0)
  constraints: 6 end point, 1 collinear, 1 perpendicular, 1 point on line
extrude "Extrusion15" add sketch "Sketch18" against normal blind 5 contours L3 L2 L1 L0 | L1 L2 L34 L18 L19 L33
thicken "Thicken1" operation add thickness 1 both sides no extend neighbours yes toward (-0.3666479, -0.9303598, 0) faces at (-67.0416, -2.4085, 1.6667)
fillet "Fillet7" radius 5 1 edges at (-56.5889, 0.8448, 2.5)
fillet "Fillet8" radius 8 1 edges at (-30.1972, -24.8028, 2.5)
sketch "Sketch19" plane through (0, 0, 0) normal (0, 0, -1) x (-1, 0, 0)
  circle A0 centre (6.2141, 68.8487) radius 2 projected
  circle A1 centre (-0.3638, 66.4546) radius 2 projected
  line L0 (-14.0502, 58.7247) -> (-16.3483, 60.653) projected
  line L1 (-16.3483, 60.653) -> (-25.9901, 49.1624) projected
  line L2 (-25.9901, 49.1624) -> (-20.6278, 44.6629) projected
  line L3 (-20.6278, 44.6629) -> (-10.986, 56.1535) projected
  arc A2 (-2.9255, 61.7976) -> (-10.986, 56.1535) centre (20.7192, 19.4516) ccw projected
  line L4 (-2.9255, 61.7976) -> (11.1699, 66.9279) projected
  line L5 (11.1699, 66.9279) -> (8.7758, 73.5057) projected
  line L6 (8.7758, 73.5057) -> (-5.3196, 68.3754) projected
  line L7 (-5.3196, 68.3754) -> (-4.2935, 65.5564) projected
  arc A3 (-4.2935, 65.5564) -> (-14.0502, 58.7247) centre (20.7465, 19.4126) ccw projected
  circle A4 centre (71.2839, 4.1003) radius 2.05 projected
  line L8 (18.7922, 50.612) -> (6.7479, 62.6632) projected
  line L9 (6.7479, 62.6632) -> (-24.8028, 30.1972) projected
  line L10 (-24.8028, 30.1972) -> (-34.8028, 30.1972) projected
  line L11 (-34.8028, 30.1972) -> (-34.8028, 10.1972) projected
  line L12 (-34.8028, 10.1972) -> (-29.0502, 10.1972) projected
  arc A5 (-25.3547, 7.7279) -> (-29.0502, 10.1972) centre (-29.0502, 6.1972) ccw projected
  line L13 (-25.3547, 7.7279) -> (-20.83, -3.1958) projected
  arc A6 (-21.6971, -7.5549) -> (-20.83, -3.1958) centre (-24.5255, -4.7265) ccw projected
  line L14 (-21.6971, -7.5549) -> (-25.7648, -11.6226) projected
  line L15 (-25.7648, -11.6226) -> (-11.6226, -25.7648) projected
  line L16 (-11.6226, -25.7648) -> (-7.5549, -21.6971) projected
  arc A7 (-3.1958, -20.83) -> (-7.5549, -21.6971) centre (-4.7265, -24.5255) ccw projected
  line L17 (-3.1958, -20.83) -> (7.7279, -25.3547) projected
  arc A8 (10.1972, -29.0502) -> (7.7279, -25.3547) centre (6.1972, -29.0502) ccw projected
  line L18 (10.1972, -29.0502) -> (10.1972, -34.8028) projected
  line L19 (10.1972, -34.8028) -> (30.1972, -34.8028) projected
  line L20 (30.1972, -34.8028) -> (30.1972, -28.1837) projected
  arc A9 (32.6218, -22.4466) -> (30.1972, -28.1837) centre (38.1972, -28.1837) ccw projected
  line L21 (32.6218, -22.4466) -> (53.0032, -2.6398) projected
  arc A10 (60.0735, -2.7409) -> (53.0032, -2.6398) centre (56.4878, -6.2256) ccw projected
  line L22 (60.0735, -2.7409) -> (62.5248, -5.2633) projected
  line L23 (62.5248, -5.2633) -> (77.9523, 0.8165) projected
  line L24 (77.9523, 0.8165) -> (73.9192, 11.0505) projected
  line L25 (73.9192, 11.0505) -> (50.612, 18.7922) projected
  line L26 (50.612, 18.7922) -> (36.1071, 4.2873) projected
  arc A11 (4.2873, 36.1071) -> (36.1071, 4.2873) centre (20.1972, 20.1972) ccw projected
  line L27 (4.2873, 36.1071) -> (18.7922, 50.612) projected
  circle A12 centre (2.0841, -7.6945) radius 2.075 projected
  circle A13 centre (-7.6945, 2.0841) radius 2.075 projected
  circle A14 centre (14.9946, -12.6504) radius 2.075 projected
  circle A15 centre (-12.6504, 14.9946) radius 2.075 projected
  line L28 (-18.8014, 27.6377) -> (-12.6669, 23.6539) projected
  arc A16 (-12.8482, 20.1946) -> (-12.6669, 23.6539) centre (-13.7562, 21.9766) ccw projected
  line L29 (-12.8482, 20.1946) -> (-19.3655, 16.8739) projected
  arc A17 (-22.272, 18.5798) -> (-19.3655, 16.8739) centre (-20.2735, 18.6559) ccw projected
  arc A18 (-21.8703, 26.245) -> (-22.272, 18.5798) centre (20.1972, 20.1972) ccw projected
  arc A19 (-18.8014, 27.6377) -> (-21.8703, 26.245) centre (-19.8907, 25.9604) ccw projected
  line L30 (-18.4561, 11.1323) -> (-11.2317, 9.988) projected
  arc A20 (-9.9903, 6.754) -> (-11.2317, 9.988) centre (-11.5446, 8.0127) ccw projected
  line L31 (-9.9903, 6.754) -> (-14.5934, 1.0696) projected
  arc A21 (-17.9425, 1.4458) -> (-14.5934, 1.0696) centre (-16.1477, 2.3282) ccw projected
  arc A22 (-20.6932, 8.6117) -> (-17.9425, 1.4458) centre (20.1972, 20.1972) ccw projected
  arc A23 (-18.4561, 11.1323) -> (-20.6932, 8.6117) centre (-18.769, 9.1569) ccw projected
  line L32 (16.8739, -19.3655) -> (20.1946, -12.8482) projected
  arc A24 (23.6539, -12.6669) -> (20.1946, -12.8482) centre (21.9766, -13.7562) ccw projected
  line L33 (23.6539, -12.6669) -> (27.6377, -18.8014) projected
  arc A25 (26.245, -21.8703) -> (27.6377, -18.8014) centre (25.9604, -19.8907) ccw projected
  arc A26 (18.5798, -22.272) -> (26.245, -21.8703) centre (20.1972, 20.1972) ccw projected
  arc A27 (16.8739, -19.3655) -> (18.5798, -22.272) centre (18.6559, -20.2735) ccw projected
  line L34 (1.0696, -14.5934) -> (6.754, -9.9903) projected
  arc A28 (9.988, -11.2317) -> (6.754, -9.9903) centre (8.0127, -11.5446) ccw projected
  line L35 (9.988, -11.2317) -> (11.1323, -18.4561) projected
  arc A29 (8.6117, -20.6932) -> (11.1323, -18.4561) centre (9.1569, -18.769) ccw projected
  arc A30 (1.4458, -17.9425) -> (8.6117, -20.6932) centre (20.1972, 20.1972) ccw projected
  arc A31 (1.0696, -14.5934) -> (1.4458, -17.9425) centre (2.3282, -16.1477) ccw projected
  line L36 (-11.4273, -3.8057) -> (-4.3621, -1.9126) projected
  arc A32 (-1.9126, -4.3621) -> (-4.3621, -1.9126) centre (-3.8444, -3.8444) ccw projected
  line L37 (-1.9126, -4.3621) -> (-3.8057, -11.4273) projected
  arc A33 (-7.0183, -12.4458) -> (-3.8057, -11.4273) centre (-5.7376, -10.9097) ccw projected
  arc A34 (-12.4458, -7.0183) -> (-7.0183, -12.4458) centre (20.1972, 20.1972) ccw projected
  arc A35 (-11.4273, -3.8057) -> (-12.4458, -7.0183) centre (-10.9097, -5.7376) ccw projected
  circle A36 centre (38.4172, 1.8124) radius 1.5 projected
  circle A37 centre (1.8124, 1.8124) radius 1.5 projected
  circle A38 centre (1.8124, 38.4172) radius 1.5 projected
  circle A39 centre (-20.2698, -11.7845) radius 1.5 projected
  circle A40 centre (-11.7845, -20.2698) radius 1.5 projected
  circle A41 centre (14.1972, -31.0318) radius 1.5 projected
  circle A42 centre (-31.0318, 26.1972) radius 1.5 projected
  circle A43 centre (-31.0318, 14.1972) radius 1.5 projected
  circle A44 centre (26.1972, -31.0318) radius 1.5 projected
  line L38 (11.1699, 66.9279) -> (16.144, 53.2617)
  line L39 (18.7922, 50.612) -> (6.7479, 62.6632) projected
  line L40 (-4.2935, 65.5564) -> (-2.9255, 61.7976)
  line L41 (-2.9255, 61.7976) -> (-0.5189, 55.1856)
  line L42 (-14.0502, 58.7247) -> (-10.986, 56.1535)
  line L43 (-10.986, 56.1535) -> (-4.7023, 50.8809)
  line L44 (6.7479, 62.6632) -> (-24.8028, 30.1972) projected
  line L45 (-20.6278, 44.6629) -> (-15.1841, 40.095)
  circle A45 centre (-18.4881, 52.658) radius 2 projected
  point P0 (0, 0)
  constraints: 12 end point, 4 collinear, 4 point on line, 1 perpendicular
extrude "Extrusion16" add sketch "Sketch19" against normal blind 5 contours A0 | A1 | L42 L3 L2 L1 L0 | L7 L6 L5 L4 L40 | L43 L9 L45 L3 | L4 L38 L8 L9 L41 | A45